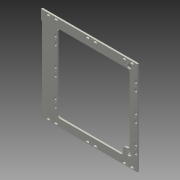
# Autodesk Inventor part: lewa_gt2
Saved by Autodesk Inventor 2013 (Build 170138000, 138)
## iProperties
Created: 2014-01-08
Part Number: lewa_gt2
Material: Generic
Document SubType Name: Modeling
Designer: dzban
Density: 1 g/cm^3
Author: dzban
Autodesk Inventor part; units mm, degrees
ref_plane "YZ Plane" through (0, 0, 0) normal (1, 0, 0) x (0, 1, 0)
ref_plane "XZ Plane" through (0, 0, 0) normal (0, 1, 0) x (-1, 0, 0)
ref_plane "XY Plane" through (0, 0, 0) normal (0, 0, 1) x (1, 0, 0)
sketch "Sketch1" plane through (0, 0, 0) normal (0, 1, 0) x (-1, 0, 0)
  line L0 (28, -266.7) -> (28, -32.6)
  arc A0 (38, -22.6) -> (28, -32.6) centre (38, -32.6) ccw
  line L1 (38, -22.6) -> (285, -22.6)
  arc A1 (295, -32.6) -> (285, -22.6) centre (285, -32.6) ccw
  line L2 (295, -32.6) -> (295, -296.7)
  arc A2 (285, -306.7) -> (295, -296.7) centre (285, -296.7) ccw
  line L3 (285, -306.7) -> (63, -306.7)
  arc A3 (53, -296.7) -> (63, -306.7) centre (63, -296.7) ccw
  line L4 (53, -296.7) -> (53, -286.7)
  arc A4 (53, -286.7) -> (43, -276.7) centre (43, -286.7) ccw
  line L5 (43, -276.7) -> (38, -276.7)
  arc A5 (28, -266.7) -> (38, -276.7) centre (38, -266.7) ccw
  line L6 (304.4, -70.45) -> (304.4, -82.45)
  line L7 (304.4, -82.45) -> (298, -82.45)
  line L8 (298, -82.45) -> (298, -70.45)
  line L9 (298, -70.45) -> (304.4, -70.45)
  line L10 (304.4, -42.85) -> (304.4, -54.85)
  line L11 (304.4, -54.85) -> (298, -54.85)
  line L12 (298, -54.85) -> (298, -42.85)
  line L13 (298, -42.85) -> (304.4, -42.85)
  line L14 (304.4, -170.45) -> (304.4, -182.45)
  line L15 (304.4, -182.45) -> (298, -182.45)
  line L16 (298, -182.45) -> (298, -170.45)
  line L17 (298, -170.45) -> (304.4, -170.45)
  line L18 (304.4, -142.85) -> (304.4, -154.85)
  line L19 (304.4, -154.85) -> (298, -154.85)
  line L20 (298, -154.85) -> (298, -142.85)
  line L21 (298, -142.85) -> (304.4, -142.85)
  line L22 (304.4, -270.45) -> (304.4, -282.45)
  line L23 (304.4, -282.45) -> (298, -282.45)
  line L24 (298, -282.45) -> (298, -270.45)
  line L25 (298, -270.45) -> (304.4, -270.45)
  line L26 (304.4, -242.85) -> (304.4, -254.85)
  line L27 (304.4, -254.85) -> (298, -254.85)
  line L28 (298, -254.85) -> (298, -242.85)
  line L29 (298, -242.85) -> (304.4, -242.85)
  line L30 (9.4, -70.45) -> (9.4, -82.45)
  line L31 (9.4, -82.45) -> (3, -82.45)
  line L32 (3, -82.45) -> (3, -70.45)
  line L33 (3, -70.45) -> (9.4, -70.45)
  line L34 (9.4, -42.85) -> (9.4, -54.85)
  line L35 (9.4, -54.85) -> (3, -54.85)
  line L36 (3, -54.85) -> (3, -42.85)
  line L37 (3, -42.85) -> (9.4, -42.85)
  line L38 (9.4, -170.45) -> (9.4, -182.45)
  line L39 (9.4, -182.45) -> (3, -182.45)
  line L40 (3, -182.45) -> (3, -170.45)
  line L41 (3, -170.45) -> (9.4, -170.45)
  line L42 (9.4, -142.85) -> (9.4, -154.85)
  line L43 (9.4, -154.85) -> (3, -154.85)
  line L44 (3, -154.85) -> (3, -142.85)
  line L45 (3, -142.85) -> (9.4, -142.85)
  line L46 (9.4, -270.45) -> (9.4, -282.45)
  line L47 (9.4, -282.45) -> (3, -282.45)
  line L48 (3, -282.45) -> (3, -270.45)
  line L49 (3, -270.45) -> (9.4, -270.45)
  line L50 (9.4, -242.85) -> (9.4, -254.85)
  line L51 (9.4, -254.85) -> (3, -254.85)
  line L52 (3, -254.85) -> (3, -242.85)
  line L53 (3, -242.85) -> (9.4, -242.85)
  line L54 (42.8, -325.3) -> (54.8, -325.3)
  line L55 (54.8, -325.3) -> (54.8, -331.7)
  line L56 (54.8, -331.7) -> (42.8, -331.7)
  line L57 (42.8, -331.7) -> (42.8, -325.3)
  line L58 (15.2, -325.3) -> (27.2, -325.3)
  line L59 (27.2, -325.3) -> (27.2, -331.7)
  line L60 (27.2, -331.7) -> (15.2, -331.7)
  line L61 (15.2, -331.7) -> (15.2, -325.3)
  line L62 (177.8, -325.3) -> (189.8, -325.3)
  line L63 (189.8, -325.3) -> (189.8, -331.7)
  line L64 (189.8, -331.7) -> (177.8, -331.7)
  line L65 (177.8, -331.7) -> (177.8, -325.3)
  line L66 (150.2, -325.3) -> (162.2, -325.3)
  line L67 (162.2, -325.3) -> (162.2, -331.7)
  line L68 (162.2, -331.7) -> (150.2, -331.7)
  line L69 (150.2, -331.7) -> (150.2, -325.3)
  line L70 (322.2, -325.3) -> (334.2, -325.3)
  line L71 (334.2, -325.3) -> (334.2, -331.7)
  line L72 (334.2, -331.7) -> (322.2, -331.7)
  line L73 (322.2, -331.7) -> (322.2, -325.3)
  line L74 (294.6, -325.3) -> (306.6, -325.3)
  line L75 (306.6, -325.3) -> (306.6, -331.7)
  line L76 (306.6, -331.7) -> (294.6, -331.7)
  line L77 (294.6, -331.7) -> (294.6, -325.3)
  line L78 (306.6, 0) -> (294.6, 0)
  line L79 (294.6, 0) -> (294.6, 6.4)
  line L80 (294.6, 6.4) -> (306.6, 6.4)
  line L81 (306.6, 6.4) -> (306.6, 0)
  line L82 (334.2, 0) -> (322.2, 0)
  line L83 (322.2, 0) -> (322.2, 6.4)
  line L84 (322.2, 6.4) -> (334.2, 6.4)
  line L85 (334.2, 6.4) -> (334.2, 0)
  line L86 (162.2, 0) -> (150.2, 0)
  line L87 (150.2, 0) -> (150.2, 6.4)
  line L88 (150.2, 6.4) -> (162.2, 6.4)
  line L89 (162.2, 6.4) -> (162.2, 0)
  line L90 (189.8, 0) -> (177.8, 0)
  line L91 (177.8, 0) -> (177.8, 6.4)
  line L92 (177.8, 6.4) -> (189.8, 6.4)
  line L93 (189.8, 6.4) -> (189.8, 0)
  line L94 (27.2, 0) -> (15.2, 0)
  line L95 (15.2, 0) -> (15.2, 6.4)
  line L96 (15.2, 6.4) -> (27.2, 6.4)
  line L97 (27.2, 6.4) -> (27.2, 0)
  line L98 (54.8, 0) -> (42.8, 0)
  line L99 (42.8, 0) -> (42.8, 6.4)
  line L100 (42.8, 6.4) -> (54.8, 6.4)
  line L101 (54.8, 6.4) -> (54.8, 0)
  line L102 (354.4, -294.7) -> (351.4, -291.7)
  line L103 (351.4, -291.7) -> (351.4, -28.6)
  line L104 (351.4, -28.6) -> (354.4, -25.6)
  line L105 (354.4, -25.6) -> (354.4, 9.4)
  line L106 (354.4, 9.4) -> (0, 9.4)
  line L107 (0, 9.4) -> (0, -334.7)
  line L108 (0, -334.7) -> (354.4, -334.7)
  line L109 (354.4, -334.7) -> (354.4, -294.7)
  circle A6 centre (20, -291.3) radius 1.5
  circle A7 centre (20, -12.3) radius 1.5
  circle A8 centre (42, -12.3) radius 1.5
  circle A9 centre (42, -291.3) radius 1.5
  circle A10 centre (35, 3.2) radius 1.5
  circle A11 centre (170, 3.2) radius 1.5
  circle A12 centre (314.4, 3.2) radius 1.5
  circle A13 centre (314.4, -328.5) radius 1.5
  circle A14 centre (170, -328.5) radius 1.5
  circle A15 centre (35, -328.5) radius 1.5
  circle A16 centre (301.2, -262.65) radius 1.5
  circle A17 centre (301.2, -162.65) radius 1.5
  circle A18 centre (301.2, -62.65) radius 1.5
  circle A19 centre (6.2, -262.65) radius 1.5
  circle A20 centre (6.2, -162.65) radius 1.5
  circle A21 centre (6.2, -62.65) radius 1.5
  circle A22 centre (31, -291.3) radius 8.05
  circle A23 centre (31, -12.3) radius 8.05
  point P0 (0, 0)
  dimension "d0" = 344.1
  dimension "d2" = 354.4
  dimension "d3" = 9.4
  dimension "d4" = 0
  dimension "d5" = 3
  dimension "d6" = 35
  dimension "d7" = 135
  dimension "d8" = 40
  dimension "d9" = 6.4
  dimension "d10" = 3.2
  dimension "d11" = 12
  dimension "d12" = 7.8
  dimension "d13" = 7.8
  dimension "d14" = 12
  dimension "d15" = 12
  dimension "d16" = 7.8
  dimension "d17" = 7.8
  dimension "d18" = 12
  dimension "d19" = 12
  dimension "d20" = 7.8
  dimension "d21" = 7.8
  dimension "d22" = 12
  dimension "d23" = 135
  dimension "d24" = 144.4
  dimension "d25" = 6.4
  dimension "d26" = 3.2
  dimension "d27" = 6.2
  dimension "d28" = 35
  dimension "d29" = 3
  dimension "d30" = 6.2
  dimension "d31" = 6.4
  dimension "d32" = 3.2
  dimension "d33" = 12
  dimension "d34" = 7.8
  dimension "d35" = 7.8
  dimension "d36" = 12
  dimension "d37" = 12
  dimension "d38" = 7.8
  dimension "d39" = 7.8
  dimension "d40" = 12
  dimension "d41" = 12
  dimension "d42" = 7.8
  dimension "d43" = 7.8
  dimension "d44" = 12
  dimension "d46" = 6.2
  dimension "d47" = 100
  dimension "d48" = 100
  dimension "d49" = 53.2
  dimension "d50" = 6.4
  dimension "d51" = 3.2
  dimension "d52" = 16.1
  dimension "d53" = 11
  dimension "d54" = 11
  dimension "d55" = 21.7
  dimension "d56" = 31
  dimension "d57" = 43.4
  dimension "d58" = 28
  dimension "d59" = 32
  dimension "d60" = 56.4
  dimension "d61" = 28
  dimension "d62" = 25
  dimension "d63" = 30
  dimension "d64" = 10
  dimension "d67" = 162.65
  constraints: 220 end point, 85 parallel, 66 collinear, 24 centre point, 22 perpendicular, 21 equal radius, 12 point on circle, 12 tangent, 11 horizontal alignment, 10 vertical alignment, 1 vertical
  measures "d0" distance between parallel lines of L106 L108
  measures "d2" distance between parallel lines of L105 L107
  measures "d3" distance from line of L106 point (0, 0)
  measures "d4" distance from line of L107 point (0, 0)
  measures "d5" distance between parallel lines of L105 L103
  measures "d6" distance of L105.end L104.end
  measures "d7" angle of L105 L104
  measures "d8" distance of L102.start L108.end
  measures "d9" distance between parallel lines of L96 L94
  measures "d10" distance from line of L96 A10.centre
  measures "d11" distance between parallel lines of L97 L95
  measures "d12" distance from line of A10.centre L97
  measures "d13" distance from line of L99 A10.centre
  measures "d14" distance between parallel lines of L101 L99
  measures "d15" distance between parallel lines of L89 L87
  measures "d16" distance from line of A11.centre L89
  measures "d17" distance from line of L91 A11.centre
  measures "d18" distance between parallel lines of L93 L91
  measures "d19" distance between parallel lines of L81 L79
  measures "d20" distance from line of L81 A12.centre
  measures "d21" distance from line of L83 A12.centre
  measures "d22" distance between parallel lines of L85 L83
  measures "d23" distance of A11.centre A10.centre
  measures "d24" distance of A12.centre A11.centre
  measures "d25" distance between parallel lines of L58 L60
  measures "d26" distance from line of A15.centre L60
  measures "d27" distance from line of L106 A10.centre
  measures "d28" distance from line of L107 A10.centre
  measures "d29" diameter of A10
  measures "d30" distance from line of L108 A15.centre
  measures "d31" distance between parallel lines of L34 L36
  measures "d32" distance from line of L34 A21.centre
  measures "d33" distance between parallel lines of L37 L35
  measures "d34" distance from line of A21.centre L35
  measures "d35" distance from line of A21.centre L33
  measures "d36" distance between parallel lines of L33 L31
  measures "d37" distance between parallel lines of L45 L43
  measures "d38" distance from line of L43 A20.centre
  measures "d39" distance from line of A20.centre L41
  measures "d40" distance between parallel lines of L41 L39
  measures "d41" distance between parallel lines of L53 L51
  measures "d42" distance from line of L51 A19.centre
  measures "d43" distance from line of A19.centre L49
  measures "d44" distance between parallel lines of L49 L47
  measures "d46" distance from line of L107 A21.centre
  measures "d47" distance of A20.centre A21.centre
  measures "d48" distance of A20.centre A19.centre
  measures "d49" distance from line of L109 A17.centre
  measures "d50" distance between parallel lines of L10 L12
  measures "d51" distance from line of L10 A18.centre
  measures "d52" diameter of A23
  measures "d53" distance of A23.centre A7.centre
  measures "d54" distance of A23.centre A8.centre
  measures "d55" distance from line of L106 A23.centre
  measures "d56" distance from line of L107 A23.centre
  measures "d57" distance from line of A22.centre L108
  measures "d58" distance between parallel lines of L107 L0
  measures "d59" distance between parallel lines of L106 L1
  measures "d60" distance between parallel lines of L103 L2
  measures "d61" distance between parallel lines of L3 L108
  measures "d62" distance between parallel lines of L0 L4
  measures "d63" distance between parallel lines of L3 L5
  measures "d64" radius of A4
  measures "d67" distance from line of A20.centre L94
extrude "Extrusion1" add sketch "Sketch1" along normal blind 6
body "Solid1"
